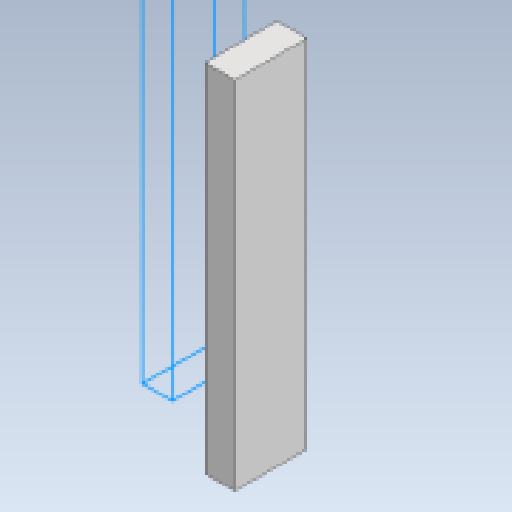
# Autodesk Inventor part: Test2
Saved by Autodesk Inventor 2025.2 (Build 292293000, 293)
## iProperties
Created: 2025-05-19
Part Number: Test2
Material: Generic
Document SubType Name: Modeling
Designer: Sergio Quintero
Density: 1.67084 g/cm^3
Appearance: Default
Mass: 12000 g
Surface Area: 3416.52 cm^2
Volume: 7182 cm^3
Author: Sergio Quintero
Autodesk Inventor part; units mm, degrees
ref_plane "YZ Plane" through (0, 0, 0) normal (1, 0, 0) x (0, 1, 0)
ref_plane "XZ Plane" through (0, 0, 0) normal (0, 1, 0) x (-1, 0, 0)
ref_plane "XY Plane" through (0, 0, 0) normal (0, 0, 1) x (1, 0, 0)
sketch "Sketch1" plane through (0, 0, 0) normal (0, 1, 0) x (-1, 0, 0)
  line L0 (-31.5, -76) -> (31.5, -76)
  line L1 (31.5, -76) -> (31.5, 76)
  line L2 (31.5, 76) -> (-31.5, 76)
  line L3 (-31.5, 76) -> (-31.5, -76)
  line L4 (-31.5, -76) -> (31.5, 76) construction
  line L5 (31.5, -76) -> (-31.5, 76) construction
  point P0 (0, 0)
  dimension "d0" = 63
  dimension "d1" = 152
  constraints: 12 end point, 2 midpoint, 2 parallel, 1 horizontal, 1 perpendicular
  measures "d0" distance of L2.end L1.end
  measures "d1" distance of L1.end L0.end
extrude "Extrusion1" add sketch "Sketch1" along normal blind 750
body "Solid1"
